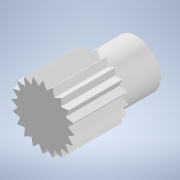
# Autodesk Inventor part: PotAttachmentB10R
Saved by Autodesk Inventor 2022 (Build 260153000, 153)
## iProperties
Created: 2021-12-04
Part Number: PotAttachmentB10R
Material: Generic
Document SubType Name: Modeling
Designer: teh18
Density: 1 g/cm^3
Appearance: Default
Author: teh18
Autodesk Inventor part; units mm, degrees
ref_plane "YZ Plane" through (0, 0, 0) normal (1, 0, 0) x (0, 1, 0)
ref_plane "XZ Plane" through (0, 0, 0) normal (0, 1, 0) x (-1, 0, 0)
ref_plane "XY Plane" through (0, 0, 0) normal (0, 0, 1) x (1, 0, 0)
ref_plane "Work Plane1" through (-2.5858, -0.1842, 12) normal (0, 0, 1) x (1, 0, 0)
sketch "Sketch1" plane through (0, 0, 0) normal (0, 0, 1) x (1, 0, 0)
  line L0 (-1.7235, 1.3627) -> (-1.9283, 2.2145) projected
  arc A0 (-1.9283, 2.2145) -> (-2.598, 1.4164) centre (0.0001, -0.0836) ccw projected
  line L1 (-2.598, 1.4164) -> (-1.7235, 1.3627) projected
  line L2 (-1.1249, 1.865) -> (-1.026, 2.7355) projected
  arc A1 (-1.026, 2.7355) -> (-1.9283, 2.2145) centre (0.0001, -0.0836) ccw projected
  line L3 (-1.9283, 2.2145) -> (-1.1249, 1.865) projected
  line L4 (-0.3906, 2.1322) -> (0.0001, 2.9164) projected
  arc A2 (0.0001, 2.9164) -> (-1.026, 2.7355) centre (0.0001, -0.0836) ccw projected
  line L5 (-1.026, 2.7355) -> (-0.3906, 2.1322) projected
  line L6 (0.3908, 2.1322) -> (1.0261, 2.7355) projected
  arc A3 (1.0261, 2.7355) -> (0.0001, 2.9164) centre (0.0001, -0.0836) ccw projected
  line L7 (0.0001, 2.9164) -> (0.3908, 2.1322) projected
  line L8 (1.0261, 2.7355) -> (1.1251, 1.865) projected
  line L9 (1.1251, 1.865) -> (1.9284, 2.2145) projected
  arc A4 (1.9284, 2.2145) -> (1.0261, 2.7355) centre (0.0001, -0.0836) ccw projected
  line L10 (1.9284, 2.2145) -> (1.7237, 1.3627) projected
  line L11 (1.7237, 1.3627) -> (2.5982, 1.4164) projected
  arc A5 (2.5982, 1.4164) -> (1.9284, 2.2145) centre (0.0001, -0.0836) ccw projected
  line L12 (2.5982, 1.4164) -> (2.1144, 0.6859) projected
  line L13 (2.1144, 0.6859) -> (2.9545, 0.4373) projected
  arc A6 (2.9545, 0.4373) -> (2.5982, 1.4164) centre (0.0001, -0.0836) ccw projected
  line L14 (-2.9543, -0.6046) -> (-2.926, -0.5836) projected
  line L15 (-2.926, -0.5836) -> (2.9262, -0.5836) projected
  line L16 (2.9262, -0.5836) -> (2.9545, -0.6046) projected
  arc A7 (2.9545, -0.6046) -> (2.9545, 0.4373) centre (0.0001, -0.0836) ccw projected
  line L17 (2.9545, 0.4373) -> (2.9262, 0.4164) projected
  line L18 (2.9262, 0.4164) -> (-2.926, 0.4164) projected
  line L19 (-2.926, 0.4164) -> (-2.9543, 0.4373) projected
  arc A8 (-2.9543, 0.4373) -> (-2.9543, -0.6046) centre (0.0001, -0.0836) ccw projected
  line L20 (2.9545, -0.6046) -> (2.1144, -0.8532) projected
  line L21 (2.1144, -0.8532) -> (2.5982, -1.5836) projected
  arc A9 (2.5982, -1.5836) -> (2.9545, -0.6046) centre (0.0001, -0.0836) ccw projected
  line L22 (2.5982, -1.5836) -> (1.7237, -1.5299) projected
  line L23 (1.7237, -1.5299) -> (1.9284, -2.3817) projected
  arc A10 (1.9284, -2.3817) -> (2.5982, -1.5836) centre (0.0001, -0.0836) ccw projected
  line L24 (1.1251, -2.0322) -> (1.0261, -2.9027) projected
  arc A11 (1.0261, -2.9027) -> (1.9284, -2.3817) centre (0.0001, -0.0836) ccw projected
  line L25 (1.9284, -2.3817) -> (1.1251, -2.0322) projected
  line L26 (0.3908, -2.2994) -> (0.0001, -3.0836) projected
  arc A12 (0.0001, -3.0836) -> (1.0261, -2.9027) centre (0.0001, -0.0836) ccw projected
  line L27 (1.0261, -2.9027) -> (0.3908, -2.2994) projected
  line L28 (-0.3906, -2.2994) -> (-1.026, -2.9027) projected
  arc A13 (-1.026, -2.9027) -> (0.0001, -3.0836) centre (0.0001, -0.0836) ccw projected
  line L29 (0.0001, -3.0836) -> (-0.3906, -2.2994) projected
  line L30 (-1.1249, -2.0322) -> (-1.9283, -2.3817) projected
  arc A14 (-1.9283, -2.3817) -> (-1.026, -2.9027) centre (0.0001, -0.0836) ccw projected
  line L31 (-1.026, -2.9027) -> (-1.1249, -2.0322) projected
  line L32 (-1.7235, -1.5299) -> (-2.598, -1.5836) projected
  arc A15 (-2.598, -1.5836) -> (-1.9283, -2.3817) centre (0.0001, -0.0836) ccw projected
  line L33 (-1.9283, -2.3817) -> (-1.7235, -1.5299) projected
  line L34 (-2.598, -1.5836) -> (-2.1142, -0.8532) projected
  line L35 (-2.1142, -0.8532) -> (-2.9543, -0.6046) projected
  arc A16 (-2.9543, -0.6046) -> (-2.598, -1.5836) centre (0.0001, -0.0836) ccw projected
  line L36 (-2.9543, 0.4373) -> (-2.1142, 0.6859) projected
  line L37 (-2.1142, 0.6859) -> (-2.598, 1.4164) projected
  arc A17 (-2.598, 1.4164) -> (-2.9543, 0.4373) centre (0.0001, -0.0836) ccw projected
  circle A18 centre (0.0001, -0.0836) radius 5
  point P0 (0, 0)
  dimension "d2" = 10
  constraints: 1 centre point, 1 coincident
  measures "d2" diameter of A18
extrude "Extrusion1" add sketch "Sketch1" along normal up to surface (12 mm away) contours L19 L18 L17 A7 L16 L15 L14 A8 | A18
sketch "Sketch2" plane through (0.0001, -0.0836, 12) normal (0, 0, 1) x (1, 0, 0)
  circle A0 centre (0, 0) radius 3.5
  point P0 (-0.0001, 0.0836)
  dimension "d3" = 7
  constraints: 1 centre point
  measures "d3" diameter of A0
extrude "Extrusion2" add sketch "Sketch2" along normal blind 2
sketch "Sketch3" plane through (0.0001, -0.0836, 14) normal (0, 0, 1) x (1, 0, 0)
  circle A0 centre (0, 0) radius 5 projected
  line L0 (0, -8.4641) -> (-3, -3.2679)
  line L1 (-3, -3.2679) -> (3, -3.2679)
  line L2 (3, -3.2679) -> (0, -8.4641)
  line L3 (2.6414, -8.0457) -> (-1.8175, -4.0309)
  line L4 (-1.8175, -4.0309) -> (3.8889, -2.1768)
  line L5 (3.8889, -2.1768) -> (2.6414, -8.0457)
  line L6 (5.0242, -6.8316) -> (-0.4571, -4.3912)
  line L7 (-0.4571, -4.3912) -> (4.397, -0.8645)
  line L8 (4.397, -0.8645) -> (5.0242, -6.8316)
  line L9 (6.9152, -4.9405) -> (0.9481, -4.3134)
  line L10 (0.9481, -4.3134) -> (4.4748, 0.5407)
  line L11 (4.4748, 0.5407) -> (6.9152, -4.9405)
  line L12 (8.1293, -2.5577) -> (2.2604, -3.8052)
  line L13 (2.2604, -3.8052) -> (4.1145, 1.9012)
  line L14 (4.1145, 1.9012) -> (8.1293, -2.5577)
  line L15 (8.5476, 0.0837) -> (3.3515, -2.9163)
  line L16 (3.3515, -2.9163) -> (3.3515, 3.0837)
  line L17 (3.3515, 3.0837) -> (8.5476, 0.0837)
  line L18 (8.1293, 2.7251) -> (4.1145, -1.7338)
  line L19 (4.1145, -1.7338) -> (2.2604, 3.9725)
  line L20 (2.2604, 3.9725) -> (8.1293, 2.7251)
  line L21 (6.9151, 5.1079) -> (4.4747, -0.3734)
  line L22 (4.4747, -0.3734) -> (0.948, 4.4807)
  line L23 (0.948, 4.4807) -> (6.9151, 5.1079)
  line L24 (5.0241, 6.9989) -> (4.3969, 1.0318)
  line L25 (4.3969, 1.0318) -> (-0.4572, 4.5585)
  line L26 (-0.4572, 4.5585) -> (5.0241, 6.9989)
  line L27 (2.6412, 8.213) -> (3.8887, 2.3441)
  line L28 (3.8887, 2.3441) -> (-1.8176, 4.1982)
  line L29 (-1.8176, 4.1982) -> (2.6412, 8.213)
  line L30 (-0.0002, 8.6313) -> (2.9998, 3.4352)
  line L31 (2.9998, 3.4352) -> (-3.0002, 3.4352)
  line L32 (-3.0002, 3.4352) -> (-0.0002, 8.6313)
  line L33 (-2.6415, 8.2129) -> (1.8173, 4.1982)
  line L34 (1.8173, 4.1982) -> (-3.889, 2.344)
  line L35 (-3.889, 2.344) -> (-2.6415, 8.2129)
  line L36 (-5.0244, 6.9988) -> (0.4569, 4.5584)
  line L37 (0.4569, 4.5584) -> (-4.3972, 1.0317)
  line L38 (-4.3972, 1.0317) -> (-5.0244, 6.9988)
  line L39 (-6.9154, 5.1078) -> (-0.9482, 4.4806)
  line L40 (-0.9482, 4.4806) -> (-4.4749, -0.3735)
  line L41 (-4.4749, -0.3735) -> (-6.9154, 5.1078)
  line L42 (-8.1295, 2.7249) -> (-2.2606, 3.9724)
  line L43 (-2.2606, 3.9724) -> (-4.1147, -1.7339)
  line L44 (-4.1147, -1.7339) -> (-8.1295, 2.7249)
  line L45 (-8.5478, 0.0835) -> (-3.3516, 3.0835)
  line L46 (-3.3516, 3.0835) -> (-3.3516, -2.9165)
  line L47 (-3.3516, -2.9165) -> (-8.5478, 0.0835)
  line L48 (-8.1294, -2.5579) -> (-4.1146, 1.901)
  line L49 (-4.1146, 1.901) -> (-2.2605, -3.8053)
  line L50 (-2.2605, -3.8053) -> (-8.1294, -2.5579)
  line L51 (-6.9153, -4.9407) -> (-4.4749, 0.5406)
  line L52 (-4.4749, 0.5406) -> (-0.9481, -4.3135)
  line L53 (-0.9481, -4.3135) -> (-6.9153, -4.9407)
  line L54 (-5.0242, -6.8317) -> (-4.3971, -0.8645)
  line L55 (-4.3971, -0.8645) -> (0.457, -4.3913)
  line L56 (0.457, -4.3913) -> (-5.0242, -6.8317)
  line L57 (-2.6414, -8.0458) -> (-3.8889, -2.1769)
  line L58 (-3.8889, -2.1769) -> (1.8175, -4.031)
  line L59 (1.8175, -4.031) -> (-2.6414, -8.0458)
  point P0 (-0.0001, 0.0836)
  point P1 (0, -5)
  point P2 (1.5709, -4.7512)
  point P3 (2.9881, -4.0291)
  point P4 (4.1127, -2.9044)
  point P5 (4.8347, -1.4872)
  point P6 (5.0835, 0.0837)
  point P7 (4.8347, 1.6546)
  point P8 (4.1126, 3.0717)
  point P9 (2.9879, 4.1964)
  point P10 (1.5708, 4.9184)
  point P11 (-0.0002, 5.1672)
  point P12 (-1.5711, 4.9184)
  point P13 (-2.9882, 4.1963)
  point P14 (-4.1128, 3.0716)
  point P15 (-4.8349, 1.6545)
  point P16 (-5.0837, 0.0835)
  point P17 (-4.8348, -1.4874)
  point P18 (-4.1128, -2.9045)
  point P19 (-2.9881, -4.0292)
  point P20 (-1.5709, -4.7512)
  point P21 (1.0624, -6.624)
  point P22 (3.0831, -5.9674)
  point P23 (4.8021, -4.7185)
  point P24 (6.051, -2.9995)
  point P25 (6.7075, -0.9787)
  point P26 (6.7075, 1.1461)
  point P27 (6.0509, 3.1668)
  point P28 (4.802, 4.8858)
  point P29 (3.083, 6.1347)
  point P30 (1.0622, 6.7912)
  point P31 (-1.0625, 6.7912)
  point P32 (-3.0833, 6.1346)
  point P33 (-4.8023, 4.8857)
  point P34 (-6.0511, 3.1667)
  point P35 (-6.7077, 1.1459)
  point P36 (-6.7077, -0.9789)
  point P37 (-6.0511, -2.9996)
  point P38 (-4.8021, -4.7186)
  point P39 (-3.0832, -5.9675)
  point P40 (-1.0624, -6.624)
  point P41 (1.5405, -2.9399)
  point P42 (0.5308, -3.2679)
  point P43 (-0.5309, -3.2679)
  point P44 (-1.5406, -2.9399)
  point P45 (-2.3995, -2.3158)
  point P46 (-3.0236, -1.4569)
  point P47 (-3.3516, -0.4472)
  point P48 (-3.3516, 0.6144)
  point P49 (-3.0236, 1.6241)
  point P50 (-2.3995, 2.4831)
  point P51 (-1.5406, 3.1071)
  point P52 (-0.5309, 3.4352)
  point P53 (0.5308, 3.4352)
  point P54 (1.5405, 3.1071)
  point P55 (2.3994, 2.4831)
  point P56 (3.0234, 1.6241)
  point P57 (3.3515, 0.6144)
  point P58 (3.3515, -0.4472)
  point P59 (3.0234, -1.4569)
  point P60 (2.3994, -2.3158)
  dimension "d6" = 6
  dimension "d9" = 360
  constraints: 120 end point, 2 vertical alignment, 1 horizontal alignment, 149 other
  measures "d6" distance of L0.end L1.end
extrude "Extrusion3" add sketch "Sketch3" against normal blind 8 contours A0 L11 L21 | A0 L21 L14 L18 L11 | L21 L11 L10 L22 L13 L25 L24 L14 A0 | A0 L14 L21 | L11 L18 A0 | A0 L18 L8 L7 L19 L10 L22 L21 L11 | L14 L24 A0 | A0 L24 L17 L21 L14 | L21 L17 L18 L14 | L21 L22 L10 L11 | L18 L11 L15 L8 A0 | A0 L8 L18 | L18 L14 L15 L11 | L24 L14 L13 L25 L16 L28 L27 L17 A0 | A0 L17 L24 | L24 L25 L13 L14 | L18 L17 L15 L14 | L21 L20 L18 L17 | L17 L24 L20 L21 | L8 L15 A0 | A0 L15 L5 L4 L16 L7 L19 L18 L8 | L18 L19 L7 L8 | L15 L14 L12 L11 | L11 L12 L8 L15 | L17 L27 A0 | A0 L27 L20 L24 L17 | L20 L24 L23 L21 | L10 L19 L13 L22 | L15 L8 L12 L5 A0 | A0 L5 L15 | L11 L9 L8 L12 | L27 L17 L16 L28 L19 L31 L30 L20 A0 | A0 L20 L27 | L27 L28 L16 L17 | L20 L27 L23 L24 | L13 L22 L16 L25 | L19 L7 L16 L10 | L10 L16 L13 L19 | L13 L19 L16 L22 | L5 L12 A0 | A0 L12 L2 L1 L13 L4 L16 L15 L5 | L15 L16 L4 L5 | L8 L9 L5 L12 | L20 L30 A0 | A0 L30 L23 L27 L20 | L23 L27 L26 L24 | L25 L19 L28 L16 | L16 L22 L19 L25 | L16 L7 L13 L10 | L10 L13 L16 | L13 L16 L19 | L16 L19 L22 | L12 L5 L9 L2 A0 | A0 L2 L12 | L8 L6 L5 L9 | L16 L4 L13 L7 | L30 L20 L19 L31 L22 L34 L33 L23 A0 | A0 L23 L30 | L30 L31 L19 L20 | L23 L30 L26 L27 | L25 L22 L28 L19 | L19 L22 L25 | L13 L7 L10 | L2 L9 A0 | A0 L9 L59 L58 L10 L1 L13 L12 L2 | L12 L13 L1 L2 | L5 L6 L2 L9 | L13 L4 L10 L7 | L23 L33 A0 | A0 L33 L26 L30 L23 | L26 L30 L29 L27 | L28 L22 L31 L19 | L25 L28 L22 | L10 L4 L7 | L9 L2 L6 L59 A0 | A0 L59 L9 | L5 L3 L2 L6 | L13 L1 L10 L4 | L33 L23 L22 L34 L25 L37 L36 L26 A0 | A0 L26 L33 | L33 L34 L22 L23 | L26 L33 L29 L30 | L28 L25 L31 L22 | L28 L31 L25 | L7 L1 L4 | L4 L10 L1 L7 | L59 L6 A0 | A0 L6 L56 L55 L7 L58 L10 L9 L59 | L9 L10 L58 L59 | L2 L3 L59 L6 | L26 L36 A0 | A0 L36 L29 L33 L26 | L29 L33 L32 L30 | L31 L25 L34 L22 | L31 L28 L34 L25 | L31 L34 L28 | L4 L58 L1 | L1 L7 L58 L4 | L1 L10 L58 L7 | L6 L59 L3 L56 A0 | A0 L56 L6 | L2 L0 L59 L3 | L36 L26 L25 L37 L28 L40 L39 L29 A0 | A0 L29 L36 | L36 L37 L25 L26 | L29 L36 L32 L33 | L34 L28 L37 L25 | L34 L31 L37 L28 | L34 L37 L31 | L58 L4 L55 L1 | L1 L55 L58 | L58 L7 L55 L4 | L56 L3 A0 | A0 L3 L53 L52 L4 L55 L7 L6 L56 | L6 L7 L55 L56 | L59 L0 L56 L3 | L29 L39 A0 | A0 L39 L32 L36 L29 | L32 L36 L35 L33 | L37 L31 L40 L28 | L37 L34 L40 L31 | L37 L40 L34 | L55 L4 L52 L1 | L1 L52 L58 L55 | L58 L52 L55 | L3 L56 L0 L53 A0 | A0 L53 L3 | L59 L57 L56 L0 | L39 L29 L28 L40 L31 L43 L42 L32 A0 | A0 L32 L39 | L39 L40 L28 L29 | L32 L39 L35 L36 | L40 L34 L43 L31 | L40 L37 L43 L34 | L40 L43 L37 | L52 L4 L3 L53 A0 L0 L50 L49 L1 | L1 L49 L58 L52 | L55 L49 L52 | L52 L58 L49 L55 | L52 L53 L3 L4 | L53 L0 A0 | L56 L57 L53 L0 | L32 L42 A0 | A0 L42 L35 L39 L32 | L35 L39 L38 L36 | L43 L34 L46 L45 L35 A0 L42 L32 L31 | L31 L32 L42 L43 | L43 L37 L46 L34 | L43 L40 L46 L37 | L43 L46 L40 | L49 L50 L0 L1 | L1 L0 L50 A0 L57 L47 L46 L58 L49 | L52 L46 L49 | L49 L55 L46 L52 | L49 L58 L46 L55 | L0 L53 L57 L50 A0 | A0 L50 L0 | L56 L54 L53 L57 | A0 L35 L42 | L35 L42 L38 L39 | L46 L37 L49 L48 L38 A0 L45 L35 L34 | L34 L35 L45 L46 | L46 L40 L49 L37 | L46 L43 L49 L40 | L46 L49 L43 | L46 L52 L43 L49 | L46 L55 L43 L52 | L46 L58 L57 L47 A0 L54 L44 L43 L55 | L46 L47 L57 L58 | L50 L57 A0 | L53 L54 L50 L57 | L35 L45 A0 | A0 L45 L38 L42 L35 | L38 L42 L41 L39 | L49 L40 L52 L51 L41 A0 L48 L38 L37 | L37 L38 L48 L49 | L49 L43 L52 L40 | L43 L55 L54 L44 A0 L51 L41 L40 L52 | L43 L44 L54 L55 | L57 L50 L54 L47 A0 | A0 L47 L57 | L53 L51 L50 L54 | A0 L38 L45 | L38 L45 L41 L42 | L40 L41 L51 L52 | L47 L54 A0 | L50 L51 L47 L54 | L38 L48 A0 | A0 L48 L41 L45 L38 | L41 L45 L44 L42 | L54 A0 L44 | L54 L47 L51 L44 A0 | L50 L48 L47 L51 | A0 L41 L48 | L41 L48 L44 L45 | L51 A0 L41 | L44 L51 A0 | L47 L48 L44 L51 | A0 L51 L44 L48 L41 | L44 L48 L47 L45
thicken "Thicken2" operation add thickness 0.2 both sides no extend neighbours yes toward (-0.8459864, -0.5332044, 0) faces at (-2.5379, -1.6832, 8)
thicken "Thicken3" operation add thickness 0.2 both sides no extend neighbours yes toward (0.96839, 0.2494411, 0) faces at (2.9052, 0.6647, 8)
body "Solid1"
